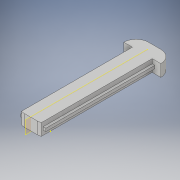
# Autodesk Inventor part: Marcus' Case Clip
Saved by Autodesk Inventor 2018 (Build 220112000, 112)
## iProperties
Created: 2019-11-26
Part Number: Marcus' Case Clip
Material: Generic
Document SubType Name: Modeling
Designer: 871357
Density: 1 g/cm^3
Appearance: Default
Author: 871357
Autodesk Inventor part; units mm, degrees
ref_plane "YZ Plane" through (0, 0, 0) normal (1, 0, 0) x (0, 1, 0)
ref_plane "XZ Plane" through (0, 0, 0) normal (0, 1, 0) x (-1, 0, 0)
ref_plane "XY Plane" through (0, 0, 0) normal (0, 0, 1) x (1, 0, 0)
sketch "Sketch1" plane through (0, 0, 0) normal (0, 1, 0) x (-1, 0, 0)
  line L0 (-6.1647, 4.8669) -> (3.9953, 4.8669)
  line L1 (3.9953, 4.8669) -> (3.9953, -52.2831)
  line L2 (3.9953, -52.2831) -> (-6.1647, -52.2831)
  line L3 (-6.1647, -52.2831) -> (-6.1647, 4.8669)
  point P0 (0, 0)
  dimension "d0" = 10.16
  dimension "d1" = 57.15
  constraints: 8 end point, 2 parallel, 1 horizontal, 1 perpendicular
  measures "d0" distance of L1.end L2.end
  measures "d1" distance of L0.end L1.end
extrude "Extrusion1" add sketch "Sketch1" along normal blind 6.096
sketch "Sketch2" plane through (6.1647, 0, 4.8669) normal (1, 0, 0) x (0, 0, -1)
  point P0 (4.8669, 0)
sketch "Sketch3" plane through (6.1647, 0, 4.8669) normal (1, 0, 0) x (0, 0, -1)
  line L0 (0, 0) -> (0, 6.096) projected
  line L1 (0, 2.286) -> (57.15, 2.286)
  line L2 (57.15, 2.286) -> (57.15, 3.81)
  line L3 (57.15, 3.81) -> (0, 3.81)
  line L4 (0, 3.81) -> (0, 2.286)
  line L5 (57.15, 0) -> (0, 0) projected
  point P0 (4.8669, 0)
  dimension "d4" = 1.524
  dimension "d5" = 57.15
  dimension "d6" = 2.286
  constraints: 8 end point, 2 parallel, 1 horizontal, 1 perpendicular, 1 point on line
  measures "d4" distance between parallel lines of L3 L1
  measures "d5" distance of L2.end L3.end
  measures "d6" distance between parallel lines of L5 L1
extrude "Extrusion2" add sketch "Sketch3" along normal blind 1.3335
ref_plane "Work Plane1" through (1.0847, 6.096, 4.8669) normal (1, 0, 0) x (0, 0, -1)
mirror "Mirror1" about plane through (1.0847, 6.096, 4.8669) normal (1, 0, 0) of "Extrusion2"
sketch "Sketch4" plane through (6.1647, 0, -52.2831) normal (0, 0, -1) x (-1, 0, 0)
  line L0 (-4.445, 0) -> (14.605, 0)
  line L1 (14.605, 0) -> (14.605, 6.096)
  line L2 (14.605, 6.096) -> (-4.445, 6.096)
  line L3 (-4.445, 6.096) -> (-4.445, 0)
  line L4 (11.4935, 2.286) -> (11.4935, 3.81) projected
  line L5 (0, 6.096) -> (10.16, 6.096) projected
  line L6 (5.08, -1.2192) -> (5.08, 7.3152) projected
  point P0 (6.1647, 0)
  dimension "d12" = 6.096
  dimension "d13" = 19.05
  dimension "d14" = 9.525
  constraints: 8 end point, 2 parallel, 1 horizontal, 1 perpendicular
  measures "d12" distance of L2.end L0.start
  measures "d13" distance of L1.end L2.end
  measures "d14" distance between parallel lines of L6 L3
extrude "Extrusion3" add sketch "Sketch4" along normal blind 6.35
fillet "Fillet2" radius 6.35 2 edges at (10.6097, 3.048, -58.6331) (-8.4403, 3.048, -58.6331)
sketch "Sketch5" plane through (0, 6.096, 0) normal (0, 1, 0) x (1, 0, 0)
  line L0 (4.2597, 58.6331) -> (-2.0903, 58.6331) projected
  line L1 (4.2597, 58.6331) -> (4.2597, -15.5891) construction
  line L2 (6.1647, -4.8669) -> (-3.9953, -4.8669) projected
  arc A0 (4.2597, -4.8669) -> (10.4219, -0.0496) centre (4.2597, 1.4831) ccw
  line L3 (11.5575, 1.4831) -> (7.7347, 1.4831) construction
  line L4 (10.4219, -0.0496) -> (12.4924, -6.8649)
  line L5 (12.4924, -6.8649) -> (5.3123, -7.0975)
  line L6 (5.3123, -7.0975) -> (4.2597, -4.8669)
  point P0 (0, 0)
  dimension "d16" = 6.35
  constraints: 10 end point, 2 line through centre, 2 point on circle, 2 point on line, 1 centre point, 1 horizontal, 1 vertical
  measures "d16" radius of A0
extrude "Extrusion4" cut sketch "Sketch5" against normal blind 7.62
mirror "Mirror2" about plane through (1.0847, 6.096, 4.8669) normal (1, 0, 0) of "Extrusion4"
sketch "Sketch6" plane through (-3.9953, 3.81, -52.2831) normal (-1, 0, 0) x (0, 0, 1)
  line L0 (55.88, 6.0179) -> (62.6058, 6.0179)
  line L1 (62.6058, 6.0179) -> (62.6058, -10.0967)
  line L2 (62.6058, -10.0967) -> (55.88, -10.0967)
  line L3 (55.88, -10.0967) -> (55.88, 6.0179)
  line L4 (0, -3.81) -> (0, 2.286) projected
  point P0 (52.2831, -3.81)
  dimension "d19" = 55.88
  constraints: 8 end point, 2 parallel, 1 horizontal, 1 perpendicular
  measures "d19" distance between parallel lines of L4 L3
extrude "Extrusion5" cut sketch "Sketch6" along normal blind 7.62
mirror "Mirror3" about plane through (1.0847, 6.096, 4.8669) normal (1, 0, 0) of "Extrusion5"
body "Solid1"
